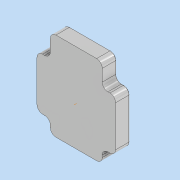
# Autodesk Inventor part: SERVO  KH56KM2U121 C
Saved by Autodesk Inventor 2021 (Build 250183000, 183)
## iProperties
Created: 2021-10-05
Part Number: SERVO  KH56KM2U121 C
Material: Generic
Document SubType Name: Modeling
Designer: 41601100
Density: 1 g/cm^3
Appearance: Default
Author: 41601100
Autodesk Inventor part; units mm, degrees
ref_plane "YZ Plane" through (0, 0, 0) normal (1, 0, 0) x (0, 1, 0)
ref_plane "XZ Plane" through (0, 0, 0) normal (0, 1, 0) x (-1, 0, 0)
ref_plane "XY Plane" through (0, 0, 0) normal (0, 0, 1) x (1, 0, 0)
sketch "Sketch1" plane through (0, 0, 0) normal (0, 0, 1) x (1, 0, 0)
  arc A0 (-24, 18.5) -> (-28, 14.5) centre (-24, 14.5) ccw
  line L0 (-28, 14.5) -> (-28, -14.5)
  arc A1 (-28, -14.5) -> (-24, -18.5) centre (-24, -14.5) ccw
  line L1 (-24, -18.5) -> (-22.5, -18.5)
  arc A2 (-18.5, -22.5) -> (-22.5, -18.5) centre (-22.5, -22.5) ccw
  line L2 (-18.5, -22.5) -> (-18.5, -24)
  arc A3 (-18.5, -24) -> (-14.5, -28) centre (-14.5, -24) ccw
  line L3 (-14.5, -28) -> (14.5, -28)
  arc A4 (14.5, -28) -> (18.5, -24) centre (14.5, -24) ccw
  line L4 (18.5, -24) -> (18.5, -22.5)
  arc A5 (22.5, -18.5) -> (18.5, -22.5) centre (22.5, -22.5) ccw
  line L5 (22.5, -18.5) -> (24, -18.5)
  arc A6 (24, -18.5) -> (28, -14.5) centre (24, -14.5) ccw
  line L6 (28, -14.5) -> (28, 14.5)
  arc A7 (28, 14.5) -> (24, 18.5) centre (24, 14.5) ccw
  line L7 (24, 18.5) -> (22.5, 18.5)
  arc A8 (18.5, 22.5) -> (22.5, 18.5) centre (22.5, 22.5) ccw
  line L8 (18.5, 22.5) -> (18.5, 24)
  line L9 (-18.5, 24) -> (-18.5, 22.5)
  arc A9 (-22.5, 18.5) -> (-18.5, 22.5) centre (-22.5, 22.5) ccw
  line L10 (-22.5, 18.5) -> (-24, 18.5)
  line L11 (0, 35) -> (-14.5, 35)
  line L12 (-18.5, 31) -> (-18.5, 24)
  line L13 (0, 35) -> (14.5, 35)
  line L14 (18.5, 31) -> (18.5, 24)
  arc A10 (-14.5, 35) -> (-18.5, 31) centre (-14.5, 31) ccw
  arc A11 (18.5, 31) -> (14.5, 35) centre (14.5, 31) ccw
  circle A12 centre (0, 0) radius 4.75
  circle A13 centre (0, 0) radius 15
  circle A14 centre (0, 0) radius 19.05
  circle A15 centre (0, 0) radius 3.15
  dimension "d1" = 4
  dimension "d4" = 9.5
  dimension "d5" = 30
  dimension "d6" = 38.1
  dimension "d7" = 6.3
  constraints: 30 end point, 24 point on circle, 16 centre point, 4 coincident, 4 tangent, 2 perpendicular, 1 equal radius, 1 horizontal
  measures "d1" radius of A10
  measures "d4" diameter of A12
  measures "d5" diameter of A13
  measures "d6" diameter of A14
  measures "d7" diameter of A15
extrude "Extrusion1" add sketch "Sketch1" along normal blind 10 contours L10 A9 L9 L12 A10 L11 L13 A11 L14 L8 A8 L7 A7 L6 A6 L5 A5 L4 A4 L3 A3 L2 A2 L1 A1 L0 A0 | A12 | A13 | A14 | A15
extrude "Extrusion2" cut sketch "Sketch1" along normal blind 2 contours A12 | A14 | A15
fillet "Fillet1" radius 0.5 27 edges at (-17.3284, 33.8284, 0) (-18.5, 26.75, 0) (-19.6716, 19.6716, 0) (-23.25, 18.5, 0) (-26.8284, 17.3284, 0) (-28, 0, 0) (-26.8284, -17.3284, 0) (-23.25, -18.5, 0) (-19.6716, -19.6716, 0) (-18.5, -23.25, 0) (-17.3284, -26.8284, 0) (0, -28, 0) (17.3284, -26.8284, 0) (18.5, -23.25, 0) (19.6716, -19.6716, 0) (23.25, -18.5, 0) (26.8284, -17.3284, 0) (28, 0, 0) (26.8284, 17.3284, 0) (23.25, 18.5, 0) (19.6716, 19.6716, 0) (18.5, 26.75, 0) (17.3284, 33.8284, 0) (0, 35, 0) (-19.05, 0, 0) (-15, 0, 0) (-4.75, 0, 0)
body "Solid1"
